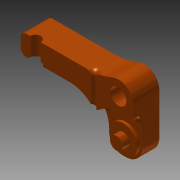
# Autodesk Inventor part: EXTRUDER ARM
Saved by Autodesk Inventor 2013 (Build 170138000, 138)
## iProperties
Created: 2014-06-22
Part Number: EXTRUDER ARM
Material: Generic
Document SubType Name: Modeling
Designer: employee
Density: 1 g/cm^3
d0: 0.189 in
d3: 0.433 in
d5: 0.829 in
d6: 0.295 in
d7: 0.984 in
d8: 0.827 in
d9: 0.386 in
d10: 0.00 deg
d12: 0.00 deg
d13: 0.787 in
d16: 0.189 in
d17: 0.098 in
d18: 0.00 deg
d19: 0.413 in
d23: 0.039 in
d24: 0.00 deg
d25: 0.079 in
d26: 0.079 in
d27: 0.157 in
d30: 0.00 deg
d31: 0.220 in
d34: 0.039 in
d35: 0.00 deg
d36: 0.079 in
d38: 0.00 deg
d39: 0.079 in
d40: 0.079 in
d43: 0.004 in
Author: employee
Autodesk Inventor part; units mm, degrees
ref_plane "YZ Plane" through (0, 0, 0) normal (1, 0, 0) x (0, 1, 0)
ref_plane "XZ Plane" through (0, 0, 0) normal (0, 1, 0) x (-1, 0, 0)
ref_plane "XY Plane" through (0, 0, 0) normal (0, 0, 1) x (1, 0, 0)
sketch "Sketch1" plane through (0, 0, 0) normal (0, 0, 1) x (1, 0, 0)
  circle A0 centre (15.5, 15.5) radius 2.9
  arc A1 (7.154059, -4.079657) -> (14.7725, -8.642004) centre (14.7725, 0) ccw
  line L0 (-18.35, 0) -> (-12.65, 0)
  line L1 (-18.35, 0) -> (-18.35, -10)
  line L2 (-18.35, -10) -> (-12.65, -10)
  line L3 (-12.65, 0) -> (-12.65, -10)
  circle A2 centre (14.7725, 0) radius 2.4
  circle A3 centre (15.5, 15.5) radius 5.5
  line L4 (15.5, 15.5) -> (21, 15.5)
  line L5 (21, 15.5) -> (21, 0)
  arc A4 (8.545, 0) -> (21, 0) centre (14.7725, 0) ccw
  arc A5 (8.545, 0) -> (-2.505, 11.05) centre (-2.505, 0) ccw
  line L6 (-2.505, 11.05) -> (-21, 11.05)
  line L7 (-21, 11.05) -> (-21, 18.55)
  line L8 (-21, 18.55) -> (3.523043, 18.55)
  arc A6 (3.523043, 18.55) -> (13.340221, 20.558197) centre (3.523043, 43.55) ccw
  circle A7 centre (15.5, 15.5) radius 3
  point P0 (0, 0)
  dimension "d0" = 4.8
  dimension "d3" = 11
  dimension "d5" = 21.05
  dimension "d6" = 7.5
  dimension "d7" = 25
  dimension "d8" = 21
  dimension "d43" = 0.1
  constraints: 10 end point, 8 point on circle, 6 centre point, 6 tangent, 3 coincident, 3 perpendicular, 2 parallel, 1 concentric, 1 horizontal alignment
  measures "d0" diameter of A2
  measures "d3" diameter of A3
  measures "d5" distance between parallel lines of L6 L2
  measures "d6" distance of L6.end L7.end
  measures "d7" radius of A6
  measures "d8" distance from line of L7 point (0, 0)
  measures "d43" radial gap between concentric circles of A7 A0
extrude "Extrusion1" add sketch "Sketch1" against normal blind 9.8 contours A2 | A3 | L5 A4 A5 L6 L7 L8 A6 A3
sketch "Sketch2" plane through (-21, 18.55, 0) normal (0, 1, 0) x (1, 0, 0)
  line L0 (24.523043, 0) -> (0, 0)
  arc A0 (7.1, 0) -> (3.9, 0) centre (5.5, 0) ccw
  line L1 (8.35, 0) -> (7.1, 0)
  line L2 (8.35, 2.85) -> (8.35, 0)
  line L3 (2.65, 2.85) -> (8.35, 2.85)
  line L4 (2.65, 0) -> (2.65, 2.85)
  line L5 (3.9, 0) -> (2.65, 0)
  point P0 (21, 0)
extrude "Extrusion2" cut sketch "Sketch2" against normal through all contours L0 A0
sketch "Sketch3" plane through (0, 0, 0) normal (0, 0, 1) x (1, 0, 0)
  arc A0 (8.545, 0) -> (21, 0) centre (14.7725, 0) ccw projected
  circle A1 centre (14.7725, 0) radius 2.4
  circle A2 centre (14.7725, 0) radius 10
  point P0 (0, 0)
  dimension "d13" = 20
  dimension "d16" = 4.8
  constraints: 2 centre point, 2 coincident
  measures "d13" diameter of A2
  measures "d16" diameter of A1
extrude "Extrusion3" cut sketch "Sketch3" against normal blind 2.5
sketch "Sketch4" plane through (0, 0, -2.5) normal (0, 0, 1) x (1, 0, 0)
  line L0 (21, 7.824209) -> (21, 0)
  arc A0 (21, 7.824209) -> (6.773382, 6.001176) centre (14.7725, 0) ccw
  arc A1 (8.545, 0) -> (6.773382, 6.001176) centre (-2.505, 0) ccw
  arc A2 (8.545, 0) -> (21, 0) centre (14.7725, 0) ccw
  circle A3 centre (14.7725, 0) radius 2.4
  circle A4 centre (14.7725, 0) radius 5.25
  point P0 (0, 0)
  dimension "d19" = 10.5
  constraints: 1 centre point, 1 coincident
  measures "d19" diameter of A4
extrude "Extrusion4" cut sketch "Sketch4" against normal blind 1 contours L0 A2 A1 A0
fillet "Fillet1" radius 2 2 edges at (21, 7.8242, -1.75) (6.7734, 6.0012, -1.75)
fillet "Fillet2" radius 2 3 edges at (20.1382, 9.5861, -3.5) (6.8068, 7.0542, -3.5) (13.0014, 9.8419, -3.5)
sketch "Sketch5" plane through (-21, 18.55, -9.8) normal (0, 1, 0) x (1, 0, 0)
  arc A0 (7.1, -9.8) -> (3.9, -9.8) centre (5.5, -9.8) ccw projected
  circle A1 centre (5.5, -9.8) radius 2
  point P0 (21, -9.8)
  dimension "d27" = 4
  constraints: 1 centre point, 1 coincident
  measures "d27" diameter of A1
extrude "Extrusion5" cut sketch "Sketch5" against normal through all
sketch "Sketch6" plane through (-21, 11.05, -9.8) normal (0, -1, 0) x (1, 0, 0)
  arc A0 (3.5, 9.8) -> (7.5, 9.8) centre (5.5, 9.8) ccw projected
  circle A1 centre (5.5, 9.8) radius 2.8
  point P0 (21, 9.8)
  dimension "d31" = 5.6
  constraints: 1 centre point, 1 coincident
  measures "d31" diameter of A1
extrude "Extrusion6" cut sketch "Sketch6" against normal blind 1
fillet "Fillet3" radius 2 2 edges at (-21, 11.05, -4.9) (-21, 18.55, -4.9)
sketch "Sketch7" plane through (3.523043, 18.55, 0) normal (0, 1, 0) x (1, 0, 0)
  circle A0 centre (2.749457, 0) radius 1.4
  circle A1 centre (2.749457, 0) radius 1
  point P0 (-3.523043, 0)
  dimension "d40" = 2
  constraints: 1 centre point, 1 coincident
  measures "d40" diameter of A1
extrude "Extrusion7" cut sketch "Sketch7" along normal through all both and the other way through all contours A1
fillet "Fillet4" radius 2 1 edges at (6.2722, 18.7016, -1)
sketch "Sketch8" plane through (0, 0, -9.8) normal (0, 0, -1) x (-1, 0, 0)
  line L0 (19, 18.55) -> (-3.523043, 18.55)
  line L1 (2.505, 11.05) -> (19, 11.05)
  line L2 (-5.2725, 7.849394) -> (-5.2725, 16.551162)
  line L3 (13.5, 18.55) -> (13.5, 12.05)
  circle A0 centre (4.11375, 14.8) radius 1.5
  line L4 (4.11375, 14.8) -> (4.11375, 18.55)
  line L5 (4.11375, 14.8) -> (4.11375, 11.05)
  line L6 (4.11375, 14.8) -> (-5.2725, 14.8)
  line L7 (4.11375, 14.8) -> (13.5, 14.8)
  point P0 (0, 0)
  dimension "d44" = 3
  constraints: 8 end point, 4 perpendicular, 4 point on line, 2 collinear, 1 centre point
  measures "d44" diameter of A0
extrude "Extrusion8" cut sketch "Sketch8" against normal through all contours L4 L6 A0 | A0 L7 L4 | A0 L5 L7 | L6 L5 A0
body "Solid1"
